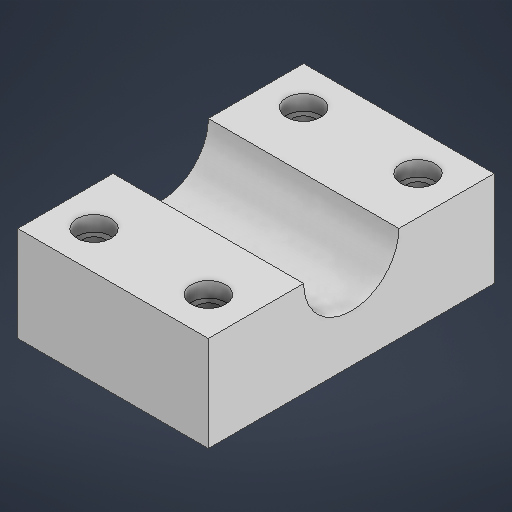
# Autodesk Inventor part: Partdia16
Saved by Autodesk Inventor 2026 (Build 300175050, 175E)
## iProperties
Created: 2026-04-16
Part Number: Partdia16
Material: Generic
Document SubType Name: Modeling
Designer: Administrator
Density: 1 g/cm^3
Appearance: Default
Author: Administrator
Autodesk Inventor part; units mm, degrees
ref_plane "YZ Plane" through (0, 0, 0) normal (1, 0, 0) x (0, 1, 0)
ref_plane "XZ Plane" through (0, 0, 0) normal (0, 1, 0) x (-1, 0, 0)
ref_plane "XY Plane" through (0, 0, 0) normal (0, 0, 1) x (1, 0, 0)
sketch "Sketch1" plane through (0, 0, 0) normal (1, 0, 0) x (0, 1, 0)
  line L0 (0, 0) -> (50, 0)
  line L1 (50, -150) -> (0, -150)
  line L2 (0, -150) -> (0, 0)
  arc A0 (50, -50) -> (50, -100) centre (50, -75) ccw
  line L3 (50, 0) -> (50, -50)
  line L4 (50, -100) -> (50, -150)
  dimension "d0" = 150
  dimension "d2" = 50
  dimension "d3" = 50
  constraints: 10 end point, 3 parallel, 2 perpendicular, 2 point on circle, 1 centre point, 1 horizontal
  measures "d0" distance of L1.end L0.start
  measures "d2" distance of L0.start L0.end
  measures "d3" diameter of A0
extrude "Extrusion1" add sketch "Sketch1" along normal mid plane 100
sketch "Sketch2" plane through (-50, 50, 0) normal (0, 1, 0) x (1, 0, 0)
  circle A0 centre (20, 20) radius 6
  circle A1 centre (20, 20) radius 9
  line L0 (0, 0) -> (100, 0) projected
  line L1 (0, 0) -> (0, 50) projected
  point P0 (50, 0)
  dimension "d6" = 18
  dimension "d7" = 12
  dimension "d8" = 20
  dimension "d9" = 20
  constraints: 2 centre point, 1 coincident
  measures "d6" diameter of A1
  measures "d7" diameter of A0
  measures "d8" distance from line of A0.centre L0
  measures "d9" distance from line of A0.centre L1
extrude "Extrusion2" cut sketch "Sketch2" against normal through all contours A0
extrude "Extrusion3" cut sketch "Sketch2" against normal blind 8 contours A0 | A1
pattern_linear "Rectangular Pattern1" count 2 spacing 110 along (0, 0, -1) count 2 spacing 60 along (1, 0, 0) of "Extrusion3", "Extrusion2"
body "Solid1"
